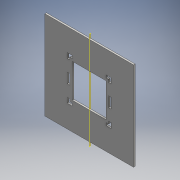
# Autodesk Inventor part: Milestone 2 Main Vehicle Chassis
Saved by Autodesk Inventor 2016 (Build 200138000, 138)
## iProperties
Created: 2016-03-09
Part Number: Milestone 2 Main Vehicle Chassis
Material: Generic
Document SubType Name: Modeling
Designer: Kenneth Daniel
Density: 1 g/cm^3
Appearance: Default
Author: Kenneth Daniel
Autodesk Inventor part; units mm, degrees
ref_plane "YZ Plane" through (0, 0, 0) normal (1, 0, 0) x (0, 1, 0)
ref_plane "XZ Plane" through (0, 0, 0) normal (0, 1, 0) x (-1, 0, 0)
ref_plane "XY Plane" through (0, 0, 0) normal (0, 0, 1) x (1, 0, 0)
sketch "Sketch1" plane through (0, 0, 0) normal (0, 1, 0) x (-1, 0, 0)
  line L0 (-175, 175) -> (-175, -175)
  line L1 (-175, -175) -> (175, -175)
  line L2 (175, -175) -> (175, 175)
  line L3 (175, 175) -> (-175, 175)
  line L4 (-175, 175) -> (175, -175) construction
  line L5 (-175, -175) -> (175, 175) construction
  line L6 (-86.5, 86.5) -> (86.5, 86.5)
  line L7 (86.5, 86.5) -> (86.5, -86.5)
  line L8 (86.5, -86.5) -> (-86.5, -86.5)
  line L9 (-86.5, -86.5) -> (-86.5, 86.5)
  line L10 (-86.5, 86.5) -> (86.5, -86.5) construction
  line L11 (86.5, 86.5) -> (-86.5, -86.5) construction
  line L12 (-66.5, 66.5) -> (-66.5, -66.5)
  line L13 (-66.5, -66.5) -> (66.5, -66.5)
  line L14 (66.5, -66.5) -> (66.5, 66.5)
  line L15 (66.5, 66.5) -> (-66.5, 66.5)
  line L16 (-66.5, 66.5) -> (66.5, -66.5) construction
  line L17 (-66.5, -66.5) -> (66.5, 66.5) construction
  line L18 (86.5, 0) -> (86.5, 20)
  line L19 (0, 233.3952) -> (0, -224.0457) construction
  line L20 (-86.5, -66.5) -> (-76.5, -66.5)
  line L21 (-76.5, -66.5) -> (-76.5, -76.5)
  line L22 (-76.5, -76.5) -> (-66.5, -76.5)
  line L23 (-66.5, -76.5) -> (-66.5, -86.5)
  line L24 (-66.5, 86.5) -> (-86.5, 86.5) construction
  line L25 (-86.5, 86.5) -> (-86.5, 66.5) construction
  line L26 (-86.5, 20) -> (-86.5, -20) construction
  line L27 (-86.5, -66.5) -> (-86.5, -86.5) construction
  line L28 (-86.5, -86.5) -> (-66.5, -86.5) construction
  point P0 (0, 0)
  dimension "d0" = 350
  dimension "d1" = 350
  dimension "d2" = 173
  dimension "d3" = 173
  dimension "d4" = 133
  dimension "d5" = 133
  constraints: 58 end point, 7 midpoint, 6 parallel, 5 collinear, 3 perpendicular, 3 vertical, 1 horizontal, 1 point on line, 1 symmetric about line
  measures "d0" distance of L0.start L0.end
  measures "d1" distance of L1.end L0.end
  measures "d2" distance of L6.start L6.end
  measures "d3" distance of L6.end L7.end
  measures "d4" distance of L12.start L12.end
  measures "d5" distance of L13.end L12.end
extrude "Extrusion1" add sketch "Sketch1" along normal blind 6.35 contours L3 L2 L1 L0 | L6 L7 L8 L23 L22 L21 L20 L9 | L20 L21 L22 L23 L8 L9
sketch "Sketch2" plane through (0, 6.35, 0) normal (0, 1, 0) x (1, 0, 0)
  line L0 (86.5, -86.5) -> (86.5, 86.5)
  line L1 (86.5, 86.5) -> (-86.5, 86.5)
  line L2 (-86.5, 86.5) -> (-86.5, -86.5)
  line L3 (-86.5, -86.5) -> (86.5, -86.5)
  line L4 (86.5, -86.5) -> (-86.5, 86.5) construction
  line L5 (86.5, 86.5) -> (-86.5, -86.5) construction
  line L6 (-66.5, -86.5) -> (-66.5, -76.5)
  line L7 (-66.5, -76.5) -> (-76.5, -76.5)
  line L8 (-76.5, -76.5) -> (-76.5, -66.5)
  line L9 (-76.5, -66.5) -> (-86.5, -66.5)
  line L10 (-86.5, -66.5) -> (-86.5, -86.5)
  line L11 (-86.5, -86.5) -> (-66.5, -86.5)
  line L12 (-86.5, 0) -> (-86.5, -20)
  line L13 (-86.5, -20) -> (-76.5, -20)
  line L14 (-76.5, -20) -> (-76.5, 20)
  line L15 (-76.5, 20) -> (-86.5, 20)
  line L16 (-86.5, 20) -> (-86.5, 0)
  line L17 (-66.5, 86.5) -> (-66.5, 76.5)
  line L18 (-66.5, 76.5) -> (-76.5, 76.5)
  line L19 (-76.5, 76.5) -> (-76.5, 66.5)
  line L20 (-76.5, 66.5) -> (-86.5, 66.5)
  line L21 (0, -182.5609) -> (0, 182.5037) construction
  line L22 (66.5, -86.5) -> (66.5, -76.5)
  line L23 (66.5, -76.5) -> (76.5, -76.5)
  line L24 (76.5, -76.5) -> (76.5, -66.5)
  line L25 (76.5, -66.5) -> (86.5, -66.5)
  line L26 (86.5, -20) -> (76.5, -20)
  line L27 (76.5, -20) -> (76.5, 20)
  line L28 (76.5, 20) -> (86.5, 20)
  line L29 (66.5, 86.5) -> (66.5, 76.5)
  line L30 (66.5, 76.5) -> (76.5, 76.5)
  line L31 (76.5, 76.5) -> (76.5, 66.5)
  line L32 (76.5, 66.5) -> (86.5, 66.5)
  point P0 (0, 0)
  dimension "d17" = 173
  dimension "d18" = 173
  dimension "d19" = 10
  dimension "d20" = 10
  dimension "d21" = 10
  dimension "d22" = 20
  dimension "d23" = 10
  dimension "d24" = 40
  dimension "d25" = 10
  dimension "d26" = 10
  dimension "d27" = 10
  dimension "d28" = 10
  constraints: 66 end point, 18 point on line, 14 symmetric about line, 6 perpendicular, 3 midpoint, 3 vertical, 2 parallel, 1 collinear
  measures "d17" distance of L0.start L0.end
  measures "d18" distance of L1.end L0.end
  measures "d19" distance of L6.start L6.end
  measures "d20" distance of L6.end L7.end
  measures "d21" distance of L7.end L8.end
  measures "d22" distance of L12.start L12.end
  measures "d23" distance of L12.end L13.end
  measures "d24" distance of L13.end L14.end
  measures "d25" distance of L14.end L15.end
  measures "d26" distance of L17.start L17.end
  measures "d27" distance of L17.end L18.end
  measures "d28" distance of L18.end L19.end
extrude "Extrusion2" cut sketch "Sketch2" against normal blind 6.35 contours L3 L2 L9 L8 L7 L6 | L2 L15 L14 L13 | L17 L18 L19 L20 L2 L1
ref_plane "Work Plane1" through (0, 0, 175) normal (1, 0, 0) x (0, 0, -1)
mirror "Mirror1" about plane through (0, 0, 175) normal (1, 0, 0) of "Extrusion2"
ref_plane "Work Plane2" through (0, 0, 175) normal (1, 0, 0) x (0, 0, -1)
body "Solid1"
